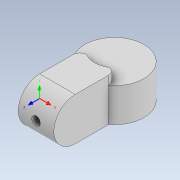
# Autodesk Inventor part: thigh_inventor
Saved by Autodesk Inventor 2020 (Build 240168000, 168)
## iProperties
Created: 2021-01-07
Part Number: thigh_inventor
Material: Generic
Document SubType Name: Modeling
Designer: DELL
Density: 1 g/cm^3
Appearance: Default
Author: DELL
Autodesk Inventor part; units mm, degrees
ref_plane "YZ Plane" through (0, 0, 0) normal (1, 0, 0) x (0, 1, 0)
ref_plane "XZ Plane" through (0, 0, 0) normal (0, 1, 0) x (-1, 0, 0)
sketch "Sketch1" plane through (0, 0, 0) normal (0, 1, 0) x (-1, 0, 0)
  line L0 (0, 0) -> (-50, 0)
  line L1 (-50, 0) -> (-50, -80)
  line L2 (-50, -80) -> (0, -80)
  line L3 (0, -80) -> (0, 0)
  circle A0 centre (-25, -80) radius 41.5
  point P0 (-50, -46.8752)
  point P1 (0, -46.8752)
  dimension "d0" = 50
  dimension "d1" = 83
  dimension "d14" = 80
  constraints: 8 end point, 2 parallel, 1 centre point, 1 horizontal, 1 midpoint, 1 perpendicular
  measures "d0" distance between parallel lines of L1 L3
  measures "d1" diameter of A0
  measures "d14" distance between parallel lines of L0 L2
extrude "Extrusion1" add sketch "Sketch1" along normal mid plane 60
sketch "Sketch2" plane through (0, 0, 0) normal (1, 0, 0) x (0, 1, 0)
  line L0 (30, 0) -> (-30, 0) projected
  circle A0 centre (0, 0) radius 30
  constraints: 1 midpoint, 3 other
extrude "Extrusion2" add sketch "Sketch2" along normal up to surface (50 mm away) contours L0 A0 picked at (-5.2341, 20.5501)
sketch "Sketch3" plane through (0, 30, 0) normal (0, 1, 0) x (1, 0, 0)
  arc A0 (50, 46.8752) -> (0, 46.8752) centre (25, 80) ccw projected
  circle A1 centre (25, 80) radius 41.5
  circle A2 centre (25, 80) radius 28
  line L0 (0, -30) -> (50, -30) construction
  line L1 (25, 80) -> (44.9219, 52.757) construction
  line L2 (8.1861, 50.8774) -> (25, 80) construction
  line L3 (50, 46.8752) -> (50, 47.5169)
  line L4 (0, 46.8752) -> (0, 0) projected
  line L5 (0, 46.8752) -> (0, 46.5678)
  circle A3 centre (25, 80) radius 33 construction
  line L6 (25, 80) -> (25, -30) construction
  line L7 (0, -30) -> (50, -30) construction
  arc A4 (11, 55.7513) -> (7.2217, 56.255) centre (8.5, 51.4212) ccw
  arc A5 (7.2217, 56.255) -> (0, 46.8752) centre (9.7022, 46.8752) ccw
  arc A6 (42.7783, 56.255) -> (39, 55.7513) centre (41.5, 51.4212) ccw
  arc A7 (50, 46.8752) -> (42.7783, 56.255) centre (40.2978, 46.8752) ccw
  point P0 (0, 46.8752)
  point P1 (66.5, 80)
  dimension "d15" = 56
  dimension "d22" = 66
  dimension "d23" = 30
  constraints: 10 end point, 8 point on circle, 4 centre point, 4 symmetric about line, 3 coincident, 2 tangent, 1 collinear, 1 midpoint, 1 point on line, 1 vertical, 12 other
  measures "d23" angle of L6 L2
extrude "Extrusion3" cut sketch "Sketch3" against normal blind 12.5 contours A7 A6 A2 A4 A5 A0 | A2
ref_plane "Work Plane1" through (25, 0, -38.5) normal (0, 0, 1) x (1, 0, 0)
sketch "Sketch4" plane through (25, 0, -38.5) normal (0, 0, 1) x (1, 0, 0)
  circle A0 centre (0, 0) radius 6
  line L0 (-14, 30) -> (14, 30) construction
  line L1 (0, 30) -> (0, -30) construction
  line L2 (-41.5, -30) -> (41.5, -30) construction
  line L3 (-25, 0) -> (25, 0) construction
  line L4 (25, -30) -> (25, 30) construction
  point P0 (-25, -30)
  point P1 (20.75, 17.5)
  point P2 (0, 0)
  dimension "d19" = 12
  constraints: 4 end point, 3 midpoint, 1 centre point, 1 coincident, 1 perpendicular, 2 other
  measures "d19" diameter of A0
extrude "Extrusion4" cut sketch "Sketch4" along normal through all
body "Solid1"
